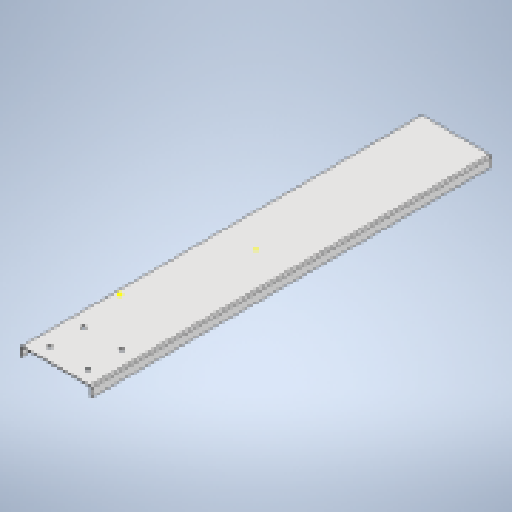
# Autodesk Inventor part: Крепление
Saved by Autodesk Inventor 2025 (Build 290162010, 162A)
## iProperties
Created: 2024-04-09
Part Number: Крепление
Material: Generic
Document SubType Name: Sheet Metal
Designer: pokla
Density: 1 g/cm^3
Sheet Metal Rule: Default_mm
Appearance: Default
Flat Pattern Width: 22.1048 cm
Flat Pattern Length: 100 cm
Flat Pattern Area: 2210.48 cm^2
Sheet Metal Width: 221,048 mm
Sheet Metal Length: 1000,000 mm
Sheet Metal Area: 221047,787 mm^2
Author: pokla
Autodesk Inventor part; units mm, degrees
ref_plane "YZ Plane" through (0, 0, 0) normal (1, 0, 0) x (0, 1, 0)
ref_plane "XZ Plane" through (0, 0, 0) normal (0, 1, 0) x (-1, 0, 0)
ref_plane "XY Plane" through (0, 0, 0) normal (0, 0, 1) x (1, 0, 0)
sketch "Sketch4" plane through (0, 0, 0) normal (0, 1, 0) x (-1, 0, 0)
  line L0 (89, -500) -> (-89, -500)
  line L1 (-89, -500) -> (-89, 500)
  line L2 (-89, 500) -> (89, 500)
  line L3 (89, 500) -> (89, -500)
  line L4 (89, -500) -> (-89, 500) construction
  point P0 (0, 0)
  point P1 (0, 0)
  dimension "d24" = 178
  dimension "d25" = 1000
  measures "d24" distance of L1.end L2.end
  measures "d25" distance of L0.end L1.end
extrude "Plate4" add sketch "Sketch4" along normal mid plane 2
sketch "Sketch7" plane through (0, -1, 0) normal (0, -1, 0) x (1, 0, 0)
  circle A0 centre (48, 382.5) radius 5
  line L0 (89, 500) -> (89, -500) projected
  line L1 (89, -500) -> (-89, -500) projected
  line L2 (0, -500) -> (0, 500) construction
  line L3 (89, 0) -> (-89, 0) construction
  circle A1 centre (-48, 382.5) radius 5
  circle A2 centre (48, 467.5) radius 5
  circle A3 centre (-48, 467.5) radius 5
  line L4 (89, 500) -> (-89, 500) projected
  point P0 (0, 0)
  point P1 (0, 0)
  dimension "d41" = 10
  dimension "d46" = 85
  dimension "d57" = 96
  dimension "d70" = 117.5
  constraints: 4 centre point, 4 end point, 4 midpoint, 2 equal radius, 2 vertical alignment, 1 coincident, 1 horizontal, 1 horizontal alignment, 1 symmetric about line, 1 vertical, 1 other
  measures "d41" diameter of A0
  measures "d46" distance of A1.centre A3.centre
  measures "d57" distance of A0.centre A1.centre
  measures "d70" distance from line of L4 A0.centre
extrude "Extrusion2" cut sketch "Sketch7" against normal up to surface (2 mm away)
sketch "Sketch9" plane through (87, 1, -500) normal (1, 0, 0) x (0, -1, 0)
  line L0 (0, 1000) -> (0, 0)
  line L1 (0, 0) -> (25, 0)
  line L2 (25, 0) -> (25, 1000)
  line L3 (25, 1000) -> (0, 1000)
  constraints: 6 end point, 1 horizontal, 1 perpendicular, 1 vertical
edge flange "Flange5" height 25 angle 90 thickness 2 bend radius 2 thickness toward (1, 0, 0) relief straight relief width 2 relief depth 1 corner gap 2 corner form 0 edges at (89, 1, 0) (-89, 1, 0) wall of the first edge with corners at (87, 1, 500) (87, 1, -500) (87, -24, -500) (87, -24, 500)
bend "Bend5"
corner "Corner5"
sketch "Sketch11" plane through (0, 1, 0) normal (0, 1, 0) x (1, 0, 0)
  circle A0 centre (-74.875, -265.5) radius 5 projected
  point P0 (0, 0)
equation "\"d24\" = Ширина_базовой_пластины"
equation "\"d25\" = Длина_базовой_пластины"
equation "\"d26\" = Thickness"
equation "\"d60\" = BendReliefWidth"
equation "\"d61\" = BendReliefDepth"
equation "\"d62\" = MinimumRemnant"
equation "\"d63\" = TransitionRadius"
equation "\"d66\" = BendRadius"
equation "\"d67\" = CornerReliefSize"
equation "\"d68\" = GapSize"
equation "\"d69\" = JacobiRadiusSize"
equation "\"BendRadius\" = Thickness"
equation "\"BendReliefWidth\" = Thickness"
equation "\"BendReliefDepth\" = 0.5 * Thickness"
equation "\"CornerReliefSize\" = 4 * Thickness"
equation "\"MinimumRemnant\" = 2 * Thickness"
equation "\"TransitionRadius\" = BendRadius"
equation "\"JacobiRadiusSize\" = BendRadius"
equation "\"GapSize\" = Thickness"
equation "\"Ширина_базовой_пластины\" = 178"
equation "\"Длина_базовой_пластины\" = 1000"
equation "\"Thickness\" = 2"
body "Solid2"
